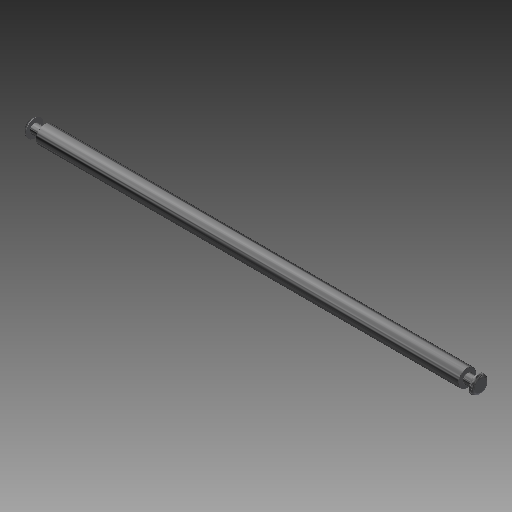
# Autodesk Inventor part: 313-01-01
Saved by Autodesk Inventor 2019 (Build 230136000, 136)
## iProperties
Company: Autodesk Inc.
Created: 2007-10-25
Part Number: 313-01-01
Document SubType Name: Modeling
Designer: Autodesk Inc.
Density: 7.85 g/cm^3
Mass: 598.597 g
Surface Area: 203.158 cm^2
Volume: 76.2544 cm^3
Material: Steel
Description: HOR SUPPORT BAR
Appearance: Rubber - Black - Version 1.1
Component Category: Lower Component
Author: Inventor
Autodesk Inventor part; units mm, degrees
ref_plane "YZ Plane" through (0, 0, 0) normal (1, 0, 0) x (0, 1, 0)
ref_plane "XZ Plane" through (0, 0, 0) normal (0, 1, 0) x (-1, 0, 0)
ref_plane "XY Plane" through (0, 0, 0) normal (0, 0, 1) x (1, 0, 0)
sketch "Sketch1" plane through (0, 0, 0) normal (0, 0, 1) x (1, 0, 0)
  line L0 (200.25, 0) -> (-200.25, 0)
  line L1 (-200.25, 0) -> (-200.25, 5.045)
  line L2 (-197.375, 7.92) -> (-197.3, 7.92)
  line L3 (-197.3, 7.92) -> (-197.3, 4.18)
  line L4 (-197.3, 4.18) -> (-188.5, 4.18)
  line L5 (-188.5, 4.18) -> (-188.5, 7.92)
  line L6 (-188.5, 7.92) -> (188.5, 7.92)
  line L7 (188.5, 7.92) -> (188.5, 4.18)
  line L8 (188.5, 4.18) -> (197.3, 4.18)
  line L9 (197.3, 4.18) -> (197.3, 7.92)
  line L10 (197.3, 7.92) -> (197.375, 7.92)
  line L11 (200.25, 5.045) -> (200.25, 0)
  arc A0 (-197.375, 7.92) -> (-200.25, 5.045) centre (-197.375, 5.045) ccw
  arc A1 (200.25, 5.045) -> (197.375, 7.92) centre (197.375, 5.045) ccw
  point P0 (0, 0)
  point P1 (0, 0)
  dimension "d0" = 400.5
  dimension "d2" = 15.84
  dimension "d4" = 8.36
  dimension "d5" = 15.84
  dimension "d7" = 8.36
  dimension "d8" = 15.84
  dimension "d15" = 2.875
  dimension "d21" = 2.95
  dimension "d22" = 8.8
  dimension "d23" = 2.95
  dimension "d24" = 8.8
  constraints: 24 end point, 7 parallel, 4 point on circle, 4 tangent, 2 centre point, 2 collinear, 2 perpendicular, 1 coincident, 1 equal radius, 1 horizontal, 1 midpoint
  measures "d0" distance of L0.start L0.end
  measures "d2" diameter of L6 L0
  measures "d4" diameter of L4 L0
  measures "d5" diameter of L2 L0
  measures "d7" diameter of L8 L0
  measures "d8" diameter of L10 L0
  measures "d15" radius of A0
  measures "d21" distance between parallel lines of L3 L1
  measures "d22" distance of L3.end L4.end
  measures "d23" distance between parallel lines of L9 L11
  measures "d24" distance of L7.end L8.end
revolve "Revolution1" add sketch "Sketch1" angle 360 about axis through (200.25, 0, 0) along (-1, 0, 0)
chamfer "Chamfer1" distance 0.375 angle 45 2 edges at (-188.5, -7.92, 0) (188.5, -7.92, 0)
fillet "Fillet1" radius 0.5 2 edges at (188.5, -4.18, 0) (-188.5, -4.18, 0)
equation "\"d7\" = d4"
equation "\"d8\" = d5"
equation "\"d24\" = d22"
body "Solid1"
